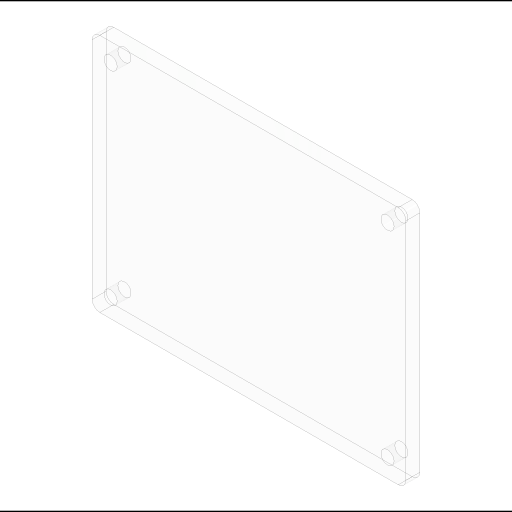
# Autodesk Inventor part: PowerBoardCaseCover
Saved by Autodesk Inventor 2023 (Build 270158000, 158)
## iProperties
Created: 2023-01-21
Part Number: PowerBoardCaseCover
Material: Polycarbonate, Clear
Document SubType Name: Modeling
Designer: kamer
Density: 1.2 g/cm^3
Appearance: Polycarbonate - Clear
Author: kamer
Autodesk Inventor part; units mm, degrees
ref_plane "YZ Plane" through (0, 0, 0) normal (1, 0, 0) x (0, 1, 0)
ref_plane "XZ Plane" through (0, 0, 0) normal (0, 1, 0) x (-1, 0, 0)
ref_plane "XY Plane" through (0, 0, 0) normal (0, 0, 1) x (1, 0, 0)
sketch "Sketch1" plane through (0, 0, 0) normal (0, 0, 1) x (1, 0, 0)
  line L0 (0, 0) -> (129.73, 0)
  line L1 (129.73, 0) -> (129.73, 99.25)
  line L2 (129.73, 99.25) -> (0, 99.25)
  line L3 (0, 99.25) -> (0, 0)
  dimension "d0" = 129.73
  dimension "d1" = 99.25
  constraints: 8 end point, 2 parallel, 1 horizontal, 1 perpendicular
  measures "d0" distance of L1.end L2.end
  measures "d1" distance of L0.end L1.end
extrude "Extrusion1" add sketch "Sketch1" along normal blind 5.7658
fillet "Fillet1" radius 3.175 4 edges at (129.73, 99.25, 2.8829) (0, 99.25, 2.8829) (0, 0, 2.8829) (129.73, 0, 2.8829)
sketch "Sketch2" plane through (0, 0, 5.7658) normal (0, 0, 1) x (1, 0, 0)
  circle A0 centre (7.62, 91.63) radius 2.7559
  circle A1 centre (122.11, 91.63) radius 2.7559
  circle A2 centre (122.11, 7.62) radius 2.7559
  circle A3 centre (7.62, 7.62) radius 2.7559
  line L0 (0, 96.075) -> (0, 3.175) projected
  line L1 (126.555, 99.25) -> (3.175, 99.25) projected
  line L2 (129.73, 3.175) -> (129.73, 96.075) projected
  line L3 (3.175, 0) -> (126.555, 0) projected
  point P0 (0, 0)
  dimension "d5" = 7.62
  dimension "d6" = 7.62
  dimension "d7" = 7.62
  dimension "d8" = 7.62
  dimension "d9" = 7.62
  dimension "d10" = 7.62
  dimension "d11" = 5.5118
  dimension "d12" = 5.5118
  dimension "d13" = 5.5118
  dimension "d14" = 7.62
  dimension "d15" = 7.62
  dimension "d16" = 5.5118
  constraints: 4 centre point
  measures "d5" distance from line of L0 A0.centre
  measures "d6" distance from line of L1 A0.centre
  measures "d7" distance from line of L1 A1.centre
  measures "d8" distance from line of L2 A1.centre
  measures "d9" distance from line of L2 A2.centre
  measures "d10" distance from line of L3 A2.centre
  measures "d11" diameter of A2
  measures "d12" diameter of A1
  measures "d13" diameter of A0
  measures "d14" distance from line of L0 A3.centre
  measures "d15" distance from line of L3 A3.centre
  measures "d16" diameter of A3
extrude "Extrusion2" cut sketch "Sketch2" against normal through all
body "Solid1"
